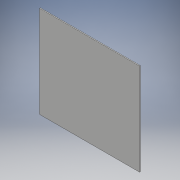
# Autodesk Inventor part: inner_panel
Saved by Autodesk Inventor 2018 (Build 220112000, 112)
## iProperties
Created: 2021-05-01
Part Number: inner_panel
Material: Generic
Document SubType Name: Modeling
Designer: gisen
Density: 1 g/cm^3
Appearance: Default
Author: gisen
Autodesk Inventor part; units mm, degrees
ref_plane "YZ Plane" through (0, 0, 0) normal (1, 0, 0) x (0, 1, 0)
ref_plane "XZ Plane" through (0, 0, 0) normal (0, 1, 0) x (-1, 0, 0)
ref_plane "XY Plane" through (0, 0, 0) normal (0, 0, 1) x (1, 0, 0)
sketch "Sketch1" plane through (0, 0, 0) normal (0, 1, 0) x (-1, 0, 0)
  line L0 (185, 170) -> (-185, 170)
  line L1 (-185, 170) -> (-185, -170)
  line L2 (-185, -170) -> (185, -170)
  line L3 (185, -170) -> (185, 170)
  line L4 (185, 170) -> (-185, -170) construction
  line L5 (-185, 170) -> (185, -170) construction
  point P0 (0, 0)
  dimension "d0" = 340
  dimension "d1" = 370
  constraints: 12 end point, 2 midpoint, 2 parallel, 1 horizontal, 1 perpendicular
  measures "d0" distance of L2.end L0.start
  measures "d1" distance of L1.end L2.end
extrude "Extrusion1" add sketch "Sketch1" along normal blind 3
body "Solid1"
